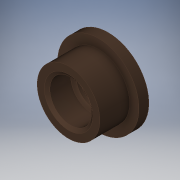
# Autodesk Inventor part: Body Cap Base Feature
Saved by Autodesk Inventor 2018 (Build 220112000, 112)
## iProperties
Created: 2017-09-07
Part Number: Body Cap Base Feature
Material: Bronze, Soft Tin
Document SubType Name: Modeling
Designer: kurtis
Density: 8.874 g/cm^3
Appearance: Bronze - Satin
Author: kurtis
Autodesk Inventor part; units mm, degrees
ref_plane "YZ Plane" through (0, 0, 0) normal (1, 0, 0) x (0, 1, 0)
ref_plane "XZ Plane" through (0, 0, 0) normal (0, 1, 0) x (-1, 0, 0)
ref_plane "XY Plane" through (0, 0, 0) normal (0, 0, 1) x (1, 0, 0)
sketch "Sketch1" plane through (0, 0, 0) normal (0, 0, 1) x (1, 0, 0)
  line L0 (0, 0) -> (28.5, 0) construction
  line L1 (28.5, 0) -> (28.5, 27)
  line L2 (0, 0) -> (19, 0) construction
  line L3 (19, 0) -> (22, 0) construction
  line L4 (28.5, 0) -> (22, 0)
  line L5 (19, 0) -> (19, 2) construction
  line L6 (19, 2) -> (22, 0)
  line L7 (19, 2) -> (19, 21)
  line L8 (19, 21) -> (16, 21) construction
  line L9 (16, 21) -> (16, 23) construction
  line L10 (16, 23) -> (19, 21)
  line L11 (16, 23) -> (16, 26)
  line L12 (16, 26) -> (20, 26)
  line L13 (20, 26) -> (20, 29)
  line L14 (20, 29) -> (25.5, 29)
  line L15 (25.5, 29) -> (25.5, 39)
  line L16 (25.5, 39) -> (28.5, 39)
  line L17 (28.5, 39) -> (28.5, 33)
  line L18 (28.5, 33) -> (33.5, 33)
  line L19 (33.5, 33) -> (33.5, 36)
  line L20 (28.5, 27) -> (37, 27)
  line L21 (37, 27) -> (37, 36)
  line L22 (37, 36) -> (33.5, 36)
  line L23 (0, 0) -> (0, 8.384) construction
  dimension "d0" = 28.5
  dimension "d1" = 27
  dimension "d2" = 19
  dimension "d3" = 3
  dimension "d4" = 2
  dimension "d5" = 21
  dimension "d6" = 3
  dimension "d7" = 2
  dimension "d8" = 3
  dimension "d17" = 3
  dimension "d18" = 5.5
  dimension "d19" = 4
  dimension "d20" = 10
  dimension "d21" = 3
  dimension "d22" = 6
  dimension "d23" = 5
  dimension "d24" = 3
  dimension "d25" = 8.5
  constraints: 48 end point, 10 perpendicular, 4 horizontal, 4 point on line, 3 vertical, 1 collinear
  measures "d0" distance of L0.start L0.end
  measures "d1" distance of L0.end L1.end
  measures "d2" distance of L0.start L2.end
  measures "d3" distance of L2.end L3.end
  measures "d4" distance of L2.end L5.end
  measures "d5" distance from line of L7.end L0
  measures "d6" distance of L7.end L8.end
  measures "d7" distance of L8.end L9.end
  measures "d8" distance of L9.end L11.end
  measures "d17" distance of L12.end L13.end
  measures "d18" distance of L13.end L14.end
  measures "d19" distance of L11.end L12.end
  measures "d20" distance of L14.end L15.end
  measures "d21" distance of L15.end L16.end
  measures "d22" distance of L16.end L17.end
  measures "d23" distance of L17.end L18.end
  measures "d24" distance of L18.end L19.end
  measures "d25" distance of L1.end L20.end
revolve "Revolution1" add sketch "Sketch1" angle 360 about axis through (0, 0, 0) along (0, 1, 0)
body "Solid1"
